OnOSwitchHolder_v2 (Autodesk Fusion 360 design; units mm, degrees)
Autodesk Fusion 360 part; units mm, degrees
sketch "Sketch1" plane through (0, 0, 0) normal (0, 0, 1) x (1, 0, 0)
  line L0 (-16, 26) -> (16, 26) construction
  line L1 (16, 26) -> (16, -26) construction
  line L2 (16, -26) -> (-16, -26) construction
  line L3 (-16, -26) -> (-16, 26) construction
  line L4 (-16, 26) -> (16, -26) construction
  line L5 (16, 26) -> (-16, -26) construction
  line L6 (-7.5, 4.3) -> (7.5, 4.3)
  line L7 (7.5, 4.3) -> (7.5, -4.3)
  line L8 (7.5, -4.3) -> (-7.5, -4.3)
  line L9 (-7.5, -4.3) -> (-7.5, 4.3)
  line L10 (-7.5, 4.3) -> (7.5, -4.3) construction
  line L11 (7.5, 4.3) -> (-7.5, -4.3) construction
  line L12 (-20, 30) -> (20, 30)
  line L13 (20, 30) -> (20, -30)
  line L14 (20, -30) -> (-20, -30)
  line L15 (-20, -30) -> (-20, 30)
  line L16 (-20, 30) -> (20, -30) construction
  line L17 (20, 30) -> (-20, -30) construction
  circle A0 centre (-16, -26) radius 1
  circle A1 centre (16, -26) radius 1
  circle A2 centre (-16, 26) radius 1
  circle A3 centre (16, 26) radius 1
  dimension "d1" = 32
  dimension "d2" = 52
  dimension "d3" = 15
  dimension "d4" = 8.6
  dimension "d5" = 40
  dimension "d6" = 60
  dimension "d7" = 2
  dimension "d8" = 2
  dimension "d9" = 2
  dimension "d10" = 2
  constraint horizontal L0
  constraint perpendicular L0 L1
  constraint parallel L0 L2
  constraint parallel L1 L3
  constraint coincident L4 origin
  constraint coincident L5 origin
  constraint horizontal L6
  constraint perpendicular L6 L7
  constraint parallel L6 L8
  constraint parallel L7 L9
  constraint coincident L10 origin
  constraint coincident L11 origin
  constraint horizontal L12
  constraint perpendicular L12 L13
  constraint parallel L12 L14
  constraint parallel L13 L15
  constraint coincident L16 origin
  constraint coincident L17 origin
  constraint coincident L2.end L3.start
  constraint coincident L1.end L2.start
  constraint coincident L0.start L3.end
  constraint coincident L0.end L1.start
  measures "d1" distance of L1.end L2.end
  measures "d2" distance of L0.end L1.end
  measures "d3" distance of L7.end L8.end
  measures "d4" distance of L6.end L7.end
  measures "d5" distance of L13.end L14.end
  measures "d6" distance of L12.end L13.end
  measures "d7" diameter of A0
  measures "d8" diameter of A1
  measures "d9" diameter of A2
  measures "d10" diameter of A3
extrude "Extrude1" add sketch "Sketch1" along normal blind 3.175
